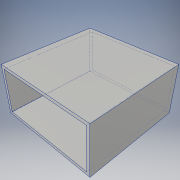
# Autodesk Inventor part: Arm 4 inch
Saved by Autodesk Inventor 2019 (Build 230136000, 136)
## iProperties
Created: 2018-09-22
Part Number: Arm 4 inch
Material: Aluminum 6061
Document SubType Name: Modeling
Designer: Adhik
Density: 2.7 g/cm^3
Appearance: Aluminum - Flat
Mass: 246.398 g
Surface Area: 602.146 cm^2
Volume: 91.2586 cm^3
Author: Adhik
Autodesk Inventor part; units mm, degrees
ref_plane "YZ Plane" through (0, 0, 0) normal (1, 0, 0) x (0, 1, 0)
ref_plane "XZ Plane" through (0, 0, 0) normal (0, 1, 0) x (-1, 0, 0)
ref_plane "XY Plane" through (0, 0, 0) normal (0, 0, 1) x (1, 0, 0)
sketch "Sketch1" plane through (0, 0, 0) normal (0, 0, 1) x (1, 0, 0)
  line L0 (-71.12, 0) -> (71.12, 0) construction
  line L1 (0, -35.56) -> (0, 35.56) construction
  line L2 (-50.8, 25.4) -> (50.8, 25.4)
  line L3 (50.8, 25.4) -> (50.8, -25.4)
  line L4 (50.8, -25.4) -> (-50.8, -25.4)
  line L5 (-50.8, -25.4) -> (-50.8, 25.4)
  line L6 (-47.625, 22.225) -> (47.625, 22.225)
  line L7 (47.625, 22.225) -> (47.625, -22.225)
  line L8 (47.625, -22.225) -> (-47.625, -22.225)
  line L9 (-47.625, -22.225) -> (-47.625, 22.225)
  point P0 (0, 0)
  point P1 (-50.8, 0)
  point P2 (0, 25.4)
  point P3 (-47.625, 0)
  point P4 (0, 22.225)
  dimension "d0" = 50.8
  dimension "d1" = 3.175
  dimension "d11" = 101.6
  dimension "d12" = 3.175
  constraints: 16 end point, 4 midpoint, 4 parallel, 4 point on line, 2 horizontal, 2 perpendicular
  measures "d0" distance of L4.end L2.start
  measures "d1" distance between parallel lines of L2 L6
  measures "d11" distance of L2.start L2.end
  measures "d12" distance between parallel lines of L5 L9
extrude "Extrusion1" add sketch "Sketch1" along normal mid plane 101.6
equation "\"d12\" = d1"
body "Solid1"
